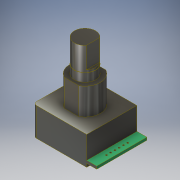
# Autodesk Inventor part: C14D32P-A3_Encoder
Saved by Autodesk Inventor 2016 (Build 200138000, 138)
## iProperties
Created: 2016-09-06
Part Number: C14D32P-A3_Encoder
Material: Generic
Document SubType Name: Modeling
Designer: jfixelle
Density: 1 g/cm^3
Appearance: Silver
Author: jfixelle
Autodesk Inventor part; units mm, degrees
ref_plane "YZ Plane" through (0, 0, 0) normal (1, 0, 0) x (0, 1, 0)
ref_plane "XZ Plane" through (0, 0, 0) normal (0, 1, 0) x (-1, 0, 0)
ref_plane "XY Plane" through (0, 0, 0) normal (0, 0, 1) x (1, 0, 0)
sketch "Sketch1" plane through (0, 0, 0) normal (0, 1, 0) x (-1, 0, 0)
  line L0 (8, 7.5) -> (-8, 7.5)
  line L1 (-8, 7.5) -> (-8, -7.5)
  line L2 (-8, -7.5) -> (8, -7.5)
  line L3 (8, -7.5) -> (8, 7.5)
  point P0 (0, 0)
  dimension "d0" = 15
  dimension "d1" = 7.5
  dimension "d2" = 16
  dimension "d3" = 8
  constraints: 8 end point, 2 parallel, 1 horizontal, 1 perpendicular
  measures "d0" distance of L2.end L0.start
  measures "d1" distance from line of point (0, 0) L2
  measures "d2" distance of L1.end L2.end
  measures "d3" distance from line of L3 point (0, 0)
extrude "Extrusion1" add sketch "Sketch1" along normal blind 8.5
fillet "Fillet1" radius 1 2 edges at (-8, 4.25, 7.5) (-8, 4.25, -7.5)
sketch "Sketch2" plane through (8, 0, 7.5) normal (0, 0, 1) x (1, 0, 0)
  line L0 (0, 0) -> (0, 8.5) projected
  line L1 (0, 1) -> (3, 1)
  line L2 (3, 1) -> (3, 1.8)
  line L3 (3, 1.8) -> (0, 1.8)
  line L4 (0, 1.8) -> (0, 1)
  line L5 (-15, 8.5) -> (0, 8.5) projected
  line L6 (-16, 8.5) -> (-16, 0) projected
  point P0 (-8, 0)
  dimension "d7" = 0.8
  dimension "d8" = 6.7
  dimension "d9" = 19
  constraints: 8 end point, 2 parallel, 1 horizontal, 1 perpendicular, 1 point on line
  measures "d7" distance of L1.end L2.end
  measures "d8" distance between parallel lines of L5 L3
  measures "d9" distance between parallel lines of L6 L2
extrude "Extrusion2" add sketch "Sketch2" against normal blind 15
sketch "Sketch3" plane through (8, 1.8, 7.5) normal (0, 1, 0) x (1, 0, 0)
  circle A0 centre (1.6, 6.865) radius 0.25
  line L0 (0, 0) -> (0, 15) construction
  line L1 (0, 9.8681) -> (0, 6.3547)
  circle A1 centre (1.6, 8.135) radius 0.25
  circle A2 centre (1.6, 9.405) radius 0.25
  circle A3 centre (1.6, 10.675) radius 0.25
  circle A4 centre (1.6, 5.595) radius 0.25
  circle A5 centre (1.6, 4.325) radius 0.25
  point P0 (-8, 7.5)
  dimension "d12" = 0.5
  dimension "d13" = 9.6
  dimension "d15" = 0.635
  dimension "d18" = 1.27
  dimension "d25" = 1.27
  constraints: 6 centre point, 2 end point, 2 point on line, 2 vertical, 10 other
  measures "d12" diameter of A0
  measures "d13" horizontal distance of point (-8, 7.5) A0.centre
  measures "d15" vertical distance of point (-8, 7.5) A0.centre
  measures "d18" distance of A0.centre A1.centre
  measures "d25" distance of A0.centre A4.centre
extrude "Extrusion3" cut sketch "Sketch3" against normal blind 15
sketch "Sketch4" plane through (0, 8.5, 0) normal (0, 1, 0) x (1, 0, 0)
  line L0 (-2.1812, 4.05) -> (2.1812, 4.05)
  line L1 (2.1812, -4.05) -> (-2.1812, -4.05)
  arc A0 (-2.1812, 4.05) -> (-2.1812, -4.05) centre (0, 0) ccw
  arc A1 (2.1812, -4.05) -> (2.1812, 4.05) centre (0, 0) ccw
  dimension "d33" = 4.05
  dimension "d34" = 8.1
  constraints: 4 end point, 4 point on circle, 2 centre point, 1 coincident, 1 horizontal, 1 parallel
  measures "d33" distance from line of L0 point (0, 0)
  measures "d34" distance between parallel lines of L1 L0
extrude "Extrusion4" add sketch "Sketch4" along normal blind 8
sketch "Sketch5" plane through (0, 16.5, 0) normal (0, 1, 0) x (1, 0, 0)
  circle A0 centre (0, 0) radius 3.2
  dimension "d37" = 6.4
  constraints: 1 centre point, 1 coincident
  measures "d37" diameter of A0
extrude "Extrusion5" add sketch "Sketch5" along normal blind 2.5
sketch "Sketch6" plane through (0, 19, 0) normal (0, 1, 0) x (1, 0, 0)
  circle A0 centre (0, 0) radius 3.15
  dimension "d40" = 6.3
  constraints: 1 centre point, 1 coincident
  measures "d40" diameter of A0
extrude "Extrusion6" add sketch "Sketch6" along normal blind 0.65
sketch "Sketch7" plane through (0, 19.65, 0) normal (0, 1, 0) x (1, 0, 0)
  arc A0 (2.41, 2.0284) -> (2.41, -2.0284) centre (0, 0) ccw
  line L0 (2.41, -2.0284) -> (2.41, 2.0284)
  dimension "d43" = 6.3
  dimension "d44" = 5.56
  constraints: 2 end point, 2 point on circle, 1 centre point, 1 coincident, 1 vertical
  measures "d43" diameter of A0
extrude "Extrusion7" add sketch "Sketch7" along normal blind 6.35
body "Solid1"
